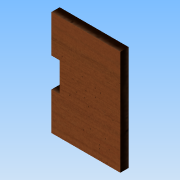
# Autodesk Inventor part: connectors
Saved by Autodesk Inventor 2015 (Build 190159000, 159)
## iProperties
Created: 2015-12-28
Part Number: connectors
Material: Générique
Document SubType Name: Modeling
Designer: Gregwar
Density: 1 g/cm^3
Appearance: Par défaut
Author: Gregwar
Autodesk Inventor part; units mm, degrees
ref_plane "YZ Plane" through (0, 0, 0) normal (1, 0, 0) x (0, 1, 0)
ref_plane "XZ Plane" through (0, 0, 0) normal (0, 1, 0) x (-1, 0, 0)
ref_plane "XY Plane" through (0, 0, 0) normal (0, 0, 1) x (1, 0, 0)
sketch "Esquisse1" plane through (0, 0, 0) normal (0, 1, 0) x (-1, 0, 0)
  line L0 (0, 0) -> (22, 0)
  line L1 (22, 0) -> (22, -32)
  line L2 (22, -32) -> (0, -32)
  line L3 (0, -32) -> (0, 0)
  dimension "d0" = 32
  dimension "d1" = 22
  constraints: 8 end point, 2 parallel, 1 horizontal, 1 perpendicular
  measures "d0" distance of L2.end L0.start
  measures "d1" distance of L0.start L0.end
extrude "Extrusion1" add sketch "Esquisse1" along normal blind 3
sketch "Esquisse2" plane through (0, 3, 0) normal (0, 1, 0) x (1, 0, 0)
  line L0 (-22, 0) -> (0, 0) projected
  line L1 (0, 0) -> (0, 32) projected
  line L2 (0, 32) -> (-22, 32) projected
  line L3 (-22, 32) -> (-22, 0) projected
  line L4 (-22, 0) -> (-25, 0)
  line L5 (-25, 0) -> (-25, 10.6667)
  line L6 (-25, 10.6667) -> (-22, 10.6667)
  line L7 (-22, 10.6667) -> (-22, 0)
  line L8 (-22, 32) -> (-25, 32)
  line L9 (-25, 32) -> (-25, 21.3333)
  line L10 (-25, 21.3333) -> (-22, 21.3333)
  line L11 (-22, 21.3333) -> (-22, 32)
  line L12 (-22, 0) -> (0, 0)
  line L13 (0, 0) -> (0, -3)
  line L14 (0, -3) -> (-22, -3)
  line L15 (-22, -3) -> (-22, 0)
  line L16 (0, 32) -> (-22, 32)
  line L17 (-22, 32) -> (-22, 35)
  line L18 (-22, 35) -> (0, 35)
  line L19 (0, 35) -> (0, 32)
  line L20 (-22, 0) -> (-25, 0)
  line L21 (-25, 0) -> (-25, -3)
  line L22 (-25, -3) -> (-22, -3)
  line L23 (-22, -3) -> (-22, 0)
  line L24 (-22, 32) -> (-25, 32)
  line L25 (-25, 32) -> (-25, 35)
  line L26 (-25, 35) -> (-22, 35)
  line L27 (-22, 35) -> (-22, 32)
  dimension "d4" = 32
  dimension "d5" = 3
  dimension "d6" = 10.6667
  dimension "d7" = 3
  constraints: 48 end point, 12 parallel, 6 horizontal, 6 perpendicular, 3 equal length, 2 point on line
  measures "d4" distance of L2.end L0.start
  measures "d5" distance of L2.end L8.end
  measures "d6" distance of L8.end L9.end
  measures "d7" distance of L14.end L0.start
extrude "Extrusion2" add sketch "Esquisse2" against normal blind 3 contours L4 L5 L6 L3 | L15 L22 L21 L4 | L0 L13 L14 L15 | L2 L17 L18 L19 | L10 L9 L8 L3 | L8 L25 L26 L17
equation "\"d6\" = 0.333333 * d4"
